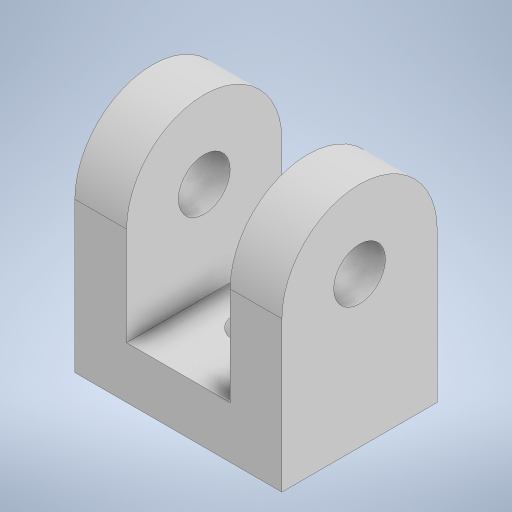
# Autodesk Inventor part: cuerpo_obj3
Saved by Autodesk Inventor 2023.2 (Build 272271030, 271C)
## iProperties
Created: 2023-02-25
Part Number: cuerpo_obj3
Material: Generic
Document SubType Name: Modeling
Designer: Cris Pat
Density: 1 g/cm^3
Appearance: Default
Author: Cris Pat
Autodesk Inventor part; units mm, degrees
ref_plane "YZ Plane" through (0, 0, 0) normal (1, 0, 0) x (0, 1, 0)
ref_plane "XZ Plane" through (0, 0, 0) normal (0, 1, 0) x (-1, 0, 0)
ref_plane "XY Plane" through (0, 0, 0) normal (0, 0, 1) x (1, 0, 0)
sketch "Sketch1" plane through (0, 0, 0) normal (1, 0, 0) x (0, 1, 0)
  line L0 (-14.5, 15) -> (-14.5, -15)
  line L1 (-14.5, -15) -> (14.5, -15)
  arc A0 (14.5, -15) -> (14.5, 15) centre (14.5, 0) ccw
  line L2 (14.5, 15) -> (-14.5, 15)
  circle A1 centre (14.5, 0) radius 5
  point P0 (0, 0)
  point P1 (0, -15)
  dimension "d0" = 15
  dimension "d1" = 10
  dimension "d2" = 29
  constraints: 6 end point, 2 centre point, 2 perpendicular, 2 point on circle, 2 vertical alignment, 1 coincident, 1 horizontal alignment, 1 midpoint, 1 tangent, 1 vertical
  measures "d0" radius of A0
  measures "d1" diameter of A1
  measures "d2" distance from line of L0 A0.centre
extrude "Extrusion1" add sketch "Sketch1" along normal mid plane 40
sketch "Sketch2" plane through (0, 0, 0) normal (0, 0, 1) x (1, 0, 0)
  line L0 (-20, 14.5) -> (20, 14.5) construction
  line L1 (20, 14.5) -> (20, 14.5) construction
  line L2 (-20, 14.5) -> (20, 14.5) construction
  line L3 (-20, 14.5) -> (-20, 14.5) construction
  line L4 (-20, 14.5) -> (20, 14.5) construction
  line L5 (20, -14.5) -> (20, 14.5) construction
  line L6 (20, -14.5) -> (-20, -14.5) construction
  line L7 (-20, 14.5) -> (-20, -14.5) construction
  line L8 (-10, 29.5) -> (10, 29.5)
  line L9 (10, 29.5) -> (10, -4.5)
  line L10 (10, -4.5) -> (-10, -4.5)
  line L11 (-10, -4.5) -> (-10, 29.5)
  line L12 (-20, 29.5) -> (20, 29.5) construction
  point P0 (0, 0)
  point P1 (0, 29.5)
  dimension "d5" = 20
  dimension "d6" = 10
  dimension "d7" = 34
  constraints: 8 end point, 2 parallel, 1 horizontal, 1 midpoint, 1 perpendicular, 1 vertical alignment
  measures "d5" distance of L9.end L10.end
  measures "d6" distance between parallel lines of L6 L10
  measures "d7" distance between parallel lines of L10 L8
extrude "Extrusion2" cut sketch "Sketch2" along normal mid plane 40
sketch "Sketch3" plane through (0, 0, 0) normal (0, 1, 0) x (-1, 0, 0)
  circle A0 centre (0, 0) radius 4.3
  dimension "d10" = 8.6
  constraints: 1 centre point, 1 coincident
  measures "d10" diameter of A0
extrude "Extrusion3" cut sketch "Sketch3" against normal through all
body "Solid1"
